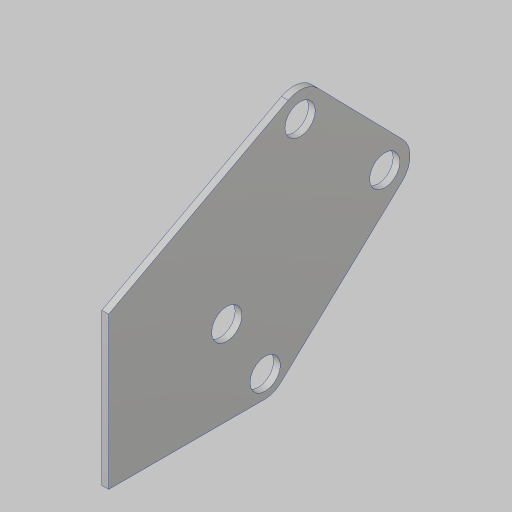
# Autodesk Inventor part: GI2 -001
Saved by Autodesk Inventor 2023.5 (Build 275446000, 446)
## iProperties
Created: 2025-01-25
Part Number: GI2 -001
Material: Aluminum 6061
Document SubType Name: Modeling
Designer: slick
Density: 2.7 g/cm^3
Appearance: Aluminum - Flat
Author: slick
Autodesk Inventor part; units mm, degrees
ref_plane "YZ Plane" through (0, 0, 0) normal (1, 0, 0) x (0, 1, 0)
ref_plane "XZ Plane" through (0, 0, 0) normal (0, 1, 0) x (-1, 0, 0)
ref_plane "XY Plane" through (0, 0, 0) normal (0, 0, 1) x (1, 0, 0)
sketch "Sketch1" plane through (0, 0, 0) normal (1, 0, 0) x (0, 1, 0)
  line L0 (0, 0) -> (50.8, 0) construction
  line L1 (50.8, 0) -> (50.8, 406.4) construction
  line L2 (50.8, 406.4) -> (0, 406.4) construction
  line L3 (0, 406.4) -> (0, 0) construction
  line L4 (-19.05, 406.4) -> (-19.05, 0) construction
  line L5 (127, 0) -> (-19.05, 0) construction
  line L6 (-19.05, 0) -> (-19.05, -76.2) construction
  line L7 (-19.05, -76.2) -> (127, -76.2) construction
  line L8 (127, -76.2) -> (127, 0) construction
  line L9 (7.9375, 127) -> (42.8625, 127) construction
  arc A0 (88.9, -76.2) -> (127, -38.1) centre (88.9, -38.1) ccw construction
  point P0 (25.4, 114.3)
  point P1 (25.4, 127)
  point P2 (25.4, 0)
  dimension "d0" = 50.8
  dimension "d1" = 406.4
  dimension "d2" = 19.05
  dimension "d3" = 146.05
  dimension "d4" = 76.2
  dimension "d5" = 34.925
  dimension "d6" = 114.3
  dimension "d7" = 12.7
  constraints: 20 end point, 5 parallel, 3 horizontal, 3 horizontal alignment, 3 midpoint, 2 perpendicular, 2 point on circle, 2 tangent, 2 vertical alignment, 1 centre point, 1 point on line, 1 vertical
  measures "d0" distance of L2.end L1.end
  measures "d1" distance of L1.end L0.end
  measures "d2" distance between parallel lines of L3 L4
  measures "d3" distance of L7.end L6.end
  measures "d4" distance of L4.end L6.end
  measures "d5" distance of L9.start L9.end
  measures "d6" distance from line of L0 point (25.4, 114.3)
  measures "d7" distance from line of point (25.4, 114.3) L9
sketch "Sketch2" plane through (0, 0, 0) normal (1, 0, 0) x (0, 1, 0)
  line L0 (0, 0) -> (50.8, 0) construction
  line L1 (50.8, 0) -> (50.8, 406.4) construction
  line L2 (50.8, 406.4) -> (0, 406.4) construction
  line L3 (0, 406.4) -> (0, 0) construction
  line L4 (-19.05, 406.4) -> (-19.05, 0) construction
  line L5 (-19.05, 0) -> (-19.05, -76.2) construction
  line L6 (7.9375, 127) -> (42.8625, 127) construction
  line L7 (127, 0) -> (-19.05, 0) construction
  line L8 (-19.05, -76.2) -> (127, -76.2) construction
  line L9 (127, -76.2) -> (127, 0) construction
  circle A0 centre (4.7625, -147.3297) radius 17.4625 construction
  circle A1 centre (63.5, -111.125) radius 25.4 construction
  circle A2 centre (38.1, -214.0803) radius 57.15 construction
  circle A3 centre (114.3, -259.8708) radius 38.1 construction
  circle A4 centre (110.5696, -171.0491) radius 57.15 construction
  circle A5 centre (63.5, -111.125) radius 19.05 construction
  circle A6 centre (195.8082, -180.1683) radius 38.1 construction
  circle A7 centre (195.8082, -180.1683) radius 28.575 construction
  circle A8 centre (114.3, -259.8708) radius 31.75 construction
  circle A9 centre (158.734, -102.8748) radius 57.15 construction
  arc A10 (88.9, -76.2) -> (127, -38.1) centre (88.9, -38.1) ccw construction
  circle A11 centre (195.8082, -180.1683) radius 14.2875
  circle A12 centre (114.3, -259.8708) radius 14.2875
  circle A13 centre (4.7625, -147.3297) radius 14.2875
  circle A14 centre (63.5, -111.125) radius 14.2875
  circle A15 centre (195.8082, -180.1683) radius 23.8125 construction
  circle A16 centre (114.3, -259.8708) radius 23.8125 construction
  circle A17 centre (4.7625, -147.3297) radius 20.6375 construction
  circle A18 centre (63.5, -111.125) radius 23.8125 construction
  line L10 (212.4565, -197.1938) -> (130.9483, -276.8963)
  line L11 (96.9036, -276.1311) -> (-10.3144, -161.422)
  line L12 (-15.875, -147.3297) -> (-15.875, 0)
  line L13 (-15.875, 0) -> (127, 0)
  line L14 (127, 0) -> (216.8344, -168.9909)
  arc A19 (96.9036, -276.1311) -> (130.9483, -276.8963) centre (114.3, -259.8708) ccw
  arc A20 (-15.875, -147.3297) -> (-10.3144, -161.422) centre (4.7625, -147.3297) ccw
  arc A21 (212.4565, -197.1938) -> (216.8344, -168.9909) centre (195.8082, -180.1683) ccw
  point P0 (25.4, 127)
  point P1 (25.4, 0)
  point P2 (25.4, 114.3)
  dimension "d8" = 34.925
  dimension "d9" = 23.8125
  dimension "d10" = 50.8
  dimension "d11" = 34.925
  dimension "d12" = 68.9991
  dimension "d13" = 82.55
  dimension "d14" = 114.3
  dimension "d15" = 76.2
  dimension "d16" = 114.3
  dimension "d17" = 6.35
  dimension "d18" = 76.2
  dimension "d19" = 9.525
  dimension "d20" = 6.35
  dimension "d21" = 114.3
  dimension "d22" = 114.0003
  dimension "d23" = 133.35
  dimension "d24" = 28.575
  dimension "d27" = 9.525
  dimension "d28" = 9.525
  dimension "d29" = 6.35
  dimension "d30" = 9.525
  constraints: 21 centre point, 14 tangent, 12 point on circle, 10 end point, 7 coincident, 4 equal radius, 1 collinear, 1 point on line, 1 vertical
  measures "d8" diameter of A0
  measures "d9" distance from line of A0.centre L5
  measures "d10" diameter of A1
  measures "d11" distance from line of A1.centre L8
  measures "d12" distance of A0.centre A1.centre
  measures "d13" distance from line of L5 A1.centre
  measures "d14" diameter of A2
  measures "d15" diameter of A3
  measures "d16" diameter of A4
  measures "d17" radial gap between concentric circles of A1 A5
  measures "d18" diameter of A6
  measures "d19" radial gap between concentric circles of A6 A7
  measures "d20" radial gap between concentric circles of A3 A8
  measures "d21" diameter of A9
  measures "d22" distance of A3.centre A6.centre
  measures "d23" distance from line of L5 A3.centre
  measures "d24" diameter of A11
  measures "d27" radial gap between concentric circles of A11 A15
  measures "d28" radial gap between concentric circles of A12 A16
  measures "d29" radial gap between concentric circles of A13 A17
  measures "d30" radial gap between concentric circles of A14 A18
extrude "Extrusion1" add sketch "Sketch2" along normal blind 6.35
body "Solid1"
